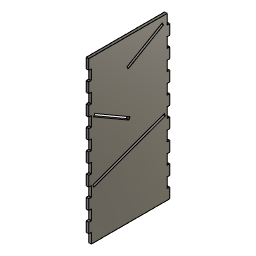
Dice Tower (Left Side) (Autodesk Fusion 360 design; units mm, degrees)
Autodesk Fusion 360 part; units mm, degrees
sketch "Sketch1" plane through (0, 0, 0) normal (1, 0, 0) x (0, 1, 0)
  line L0 (-98.425, 88.9) -> (-101.6, 88.9)
  line L1 (-98.425, 38.1) -> (-98.425, 25.4)
  line L2 (-98.425, 76.2) -> (-101.6, 76.2)
  line L3 (-101.6, 0) -> (-100.0125, 0)
  line L4 (-98.425, 190.5) -> (-98.425, 177.8)
  line L5 (-101.6, 203.2) -> (-98.425, 203.2)
  line L6 (-98.425, 177.8) -> (-98.425, 165.1)
  line L7 (-98.425, 203.2) -> (-98.425, 177.8)
  line L8 (-3.175, 177.8) -> (0, 177.8)
  line L9 (-98.425, 127) -> (-101.6, 127)
  line L10 (-3.175, 165.1) -> (0, 165.1)
  line L11 (-98.425, 165.1) -> (-98.425, 152.4)
  line L12 (0, 12.7) -> (-3.175, 12.7)
  line L13 (0, 127) -> (-3.175, 127)
  line L14 (-101.6, 76.2) -> (-101.6, 63.5)
  line L15 (-98.425, 63.5) -> (-98.425, 50.8)
  line L16 (-98.425, 114.3) -> (-98.425, 101.6)
  line L17 (-101.6, 101.6) -> (-101.6, 88.9)
  line L18 (-101.6, 0) -> (-98.425, 0)
  line L19 (-98.425, 63.5) -> (-101.6, 63.5)
  line L20 (-101.6, 0) -> (-90.5002, 0)
  line L21 (-3.175, 190.5) -> (-3.175, 177.8)
  line L22 (-3.175, 50.8) -> (0, 50.8)
  line L23 (0, 25.4) -> (-3.175, 25.4)
  line L24 (-3.175, 152.4) -> (-3.175, 139.7)
  line L25 (0, 38.1) -> (-3.175, 38.1)
  line L26 (-101.6, 177.8) -> (-101.6, 165.1)
  line L27 (0, 0) -> (-3.175, 0)
  line L28 (-3.175, 190.5) -> (0, 190.5)
  line L29 (-3.175, 50.8) -> (-3.175, 38.1)
  line L30 (-101.6, 203.2) -> (-101.6, 190.5)
  line L31 (-101.6, 127) -> (-101.6, 114.3)
  line L32 (-98.425, 114.3) -> (-101.6, 114.3)
  line L33 (0, 0) -> (-11.0998, 0)
  line L34 (-98.425, 139.7) -> (-98.425, 127)
  line L35 (-3.175, 177.8) -> (-3.175, 165.1)
  line L36 (-98.425, 165.1) -> (-101.6, 165.1)
  line L37 (-11.0998, 0) -> (-6.0198, 0)
  line L38 (0, 152.4) -> (-3.175, 152.4)
  line L39 (0, 0) -> (-12.065, 0)
  line L40 (-3.175, 76.2) -> (-3.175, 63.5)
  line L41 (-3.175, 139.7) -> (0, 139.7)
  line L42 (-3.175, 12.7) -> (-3.175, 0)
  line L43 (-90.5002, 0) -> (-95.5802, 0)
  line L44 (-98.425, 101.6) -> (-101.6, 101.6)
  line L45 (-3.175, 101.6) -> (-3.175, 88.9)
  line L46 (-3.175, 0) -> (-3.175, 59.055)
  line L47 (-3.175, 88.9) -> (-3.175, 76.2)
  line L48 (-98.425, 177.8) -> (-101.6, 177.8)
  line L49 (-3.175, 38.1) -> (-3.175, 25.4)
  line L50 (-98.425, 152.4) -> (-98.425, 139.7)
  line L51 (-98.425, 203.2) -> (-98.425, 190.5)
  line L52 (-98.425, 139.7) -> (-101.6, 139.7)
  line L53 (-3.175, 63.5) -> (0, 63.5)
  line L54 (-3.175, 203.2) -> (-3.175, 190.5)
  line L55 (-98.425, 127) -> (-98.425, 114.3)
  line L56 (-3.175, 63.5) -> (-3.175, 50.8)
  line L57 (-3.175, 88.9) -> (0, 88.9)
  line L58 (-3.175, 114.3) -> (0, 114.3)
  line L59 (0, 101.6) -> (-3.175, 101.6)
  line L60 (-3.175, 127) -> (-3.175, 114.3)
  line L61 (-98.425, 190.5) -> (-101.6, 190.5)
  line L62 (-98.425, 0) -> (-98.425, 203.2)
  line L63 (-3.175, 76.2) -> (0, 76.2)
  line L64 (-98.425, 152.4) -> (-101.6, 152.4)
  line L65 (-98.425, 25.4) -> (-98.425, 12.7)
  line L66 (-101.6, 152.4) -> (-101.6, 139.7)
  line L67 (-98.425, 38.1) -> (-101.6, 38.1)
  line L68 (-101.6, 0) -> (0, 0)
  line L69 (-98.425, 50.8) -> (-101.6, 50.8)
  line L70 (-101.6, 50.8) -> (-101.6, 38.1)
  line L71 (-98.425, 50.8) -> (-98.425, 38.1)
  line L72 (-101.6, 0) -> (-85.725, 0)
  line L73 (-3.175, 0) -> (-3.175, 203.2)
  line L74 (-98.425, 101.6) -> (-98.425, 95.25)
  line L75 (-98.425, 95.25) -> (-98.425, 88.9)
  line L76 (-3.175, 203.2) -> (-101.6, 203.2)
  line L77 (-98.425, 88.9) -> (-98.425, 76.2)
  line L78 (-3.175, 25.4) -> (-3.175, 12.7)
  line L79 (-98.425, 76.2) -> (-98.425, 63.5)
  line L80 (-101.6, 25.4) -> (-101.6, 12.7)
  line L81 (-98.425, 12.7) -> (-101.6, 12.7)
  line L82 (-98.425, 25.4) -> (-101.6, 25.4)
  line L83 (-6.8245, 95.8167) -> (-96.3434, 63.2754)
  line L84 (-53.6764, 170.2912) -> (-53.4564, 170.4182)
  line L85 (-6.5858, 95.9034) -> (-6.8245, 95.8167)
  line L86 (-51.6199, 111.4777) -> (-51.4, 111.3504)
  line L87 (-7.8589, 193.04) -> (-51.8566, 167.6463)
  line L88 (-95.5835, 136.9303) -> (-93.98, 139.7)
  line L89 (-9.4587, 195.8119) -> (-7.8589, 193.04)
  line L90 (-51.8566, 167.6463) -> (-52.0766, 167.5194)
  line L91 (-5.4924, 92.8956) -> (-6.5858, 95.9034)
  line L92 (-51.6199, 111.4777) -> (-95.5835, 136.9303)
  line L93 (-93.98, 139.7) -> (-50.0163, 114.2474)
  line L94 (-96.3434, 63.2754) -> (-95.25, 60.2676)
  line L95 (-53.4564, 170.4182) -> (-9.4587, 195.8119)
  line L96 (-5.7311, 92.8088) -> (-5.4924, 92.8956)
  line L97 (-51.4, 111.3504) -> (-49.7965, 114.1201)
  line L98 (-95.25, 60.2676) -> (-5.7311, 92.8088)
  line L99 (-49.7965, 114.1201) -> (-50.0163, 114.2474)
  line L100 (-52.0766, 167.5194) -> (-53.6764, 170.2912)
  line L101 (0, 190.5) -> (0, 177.8)
  line L102 (0, 165.1) -> (0, 152.4)
  line L103 (0, 139.7) -> (0, 127)
  line L104 (0, 114.3) -> (0, 101.6)
  line L105 (0, 88.9) -> (0, 76.2)
  line L106 (0, 63.5) -> (0, 50.8)
  line L107 (0, 38.1) -> (0, 25.4)
  line L108 (0, 12.7) -> (0, 0)
  dimension "d92" = 50.8
  dimension "d93" = 3.2004
  dimension "d94" = 50.8
  dimension "d95" = 50.8
  dimension "d96" = 3.2004
  dimension "d97" = 50.8
  dimension "d98" = 95.25
  dimension "d99" = 3.2004
  dimension "d100" = 95.25
  dimension "d101" = 0.254
  dimension "d102" = 0.254
  dimension "d103" = 3.2004
  dimension "d104" = 0.254
  dimension "d105" = 3.2004
  constraint perpendicular L92 L97
  constraint parallel L96 L98
  constraint perpendicular L91 L96
  constraint parallel L87 L90
  constraint perpendicular L90 L100
  constraint perpendicular L84 L100
  constraint perpendicular L94 L98
  constraint perpendicular L8 L101
  constraint perpendicular L38 L102
  constraint perpendicular L13 L103
  constraint perpendicular L59 L104
  constraint perpendicular L63 L105
  constraint perpendicular L22 L106
  constraint parallel L106 L107
  constraint perpendicular L27 L108
  measures "d92" distance of L88.end L93.end
  measures "d93" distance of L93.end L86.start
  measures "d94" distance of L88.start L86.start
  measures "d95" distance of L87.start L87.end
  measures "d96" distance of L84.end L87.end
  measures "d97" distance of L84.end L89.start
  measures "d98" distance of L94.end L96.start
  measures "d99" distance of L96.start L83.start
  measures "d100" distance of L83.end L83.start
  measures "d101" distance of L86.start L86.end
  measures "d102" distance of L96.start L91.start
  measures "d103" distance of L85.start L91.start
  measures "d104" distance of L90.end L87.end
  measures "d105" distance of L84.start L90.end
extrude "Extrude1" add sketch "Sketch1" along normal blind 3.175
sketch "Sketch2" plane through (0, 0, 0) normal (1, 0, 0) x (0, 1, 0)
